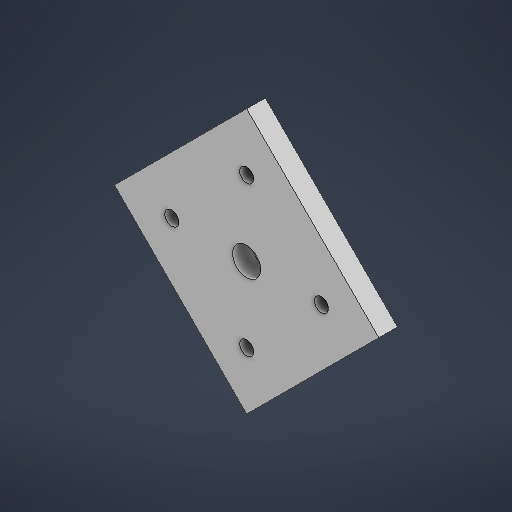
# Autodesk Inventor part: drzakmotoru_nový
Saved by Autodesk Inventor 2026 (Build 300175050, 175E)
## iProperties
Created: 2026-04-28
Part Number: drzakmotoru_nový
Material: Všeobecné
Document SubType Name: Modeling
Designer: marti
Density: 1 g/cm^3
Appearance: Výchozí
Author: marti
Autodesk Inventor part; units mm, degrees
ref_plane "YZ Plane" through (0, 0, 0) normal (1, 0, 0) x (0, 1, 0)
ref_plane "XZ Plane" through (0, 0, 0) normal (0, 1, 0) x (-1, 0, 0)
ref_plane "XY Plane" through (0, 0, 0) normal (0, 0, 1) x (1, 0, 0)
sketch "Náčrt1" plane through (0, 0, 0) normal (0, 0, 1) x (1, 0, 0)
  line L0 (-28.2843, 0) -> (0, 28.2843)
  line L1 (0, 28.2843) -> (28.2843, 0)
  line L2 (28.2843, 0) -> (0, -28.2843)
  line L3 (0, -28.2843) -> (-28.2843, 0)
  line L4 (-28.2843, 0) -> (28.2843, 0) construction
  line L5 (0, 28.2843) -> (0, -28.2843) construction
  line L6 (-28.2843, 0) -> (11.7157, 0) construction
  line L7 (0, 39.598) -> (0, -39.598) projected
  line L8 (-39.598, 0) -> (39.598, 0) projected
  point P0 (0, 0)
  point P1 (-16, 0)
  point P2 (16, 0)
  point P3 (0, 0)
  point P4 (0, 16)
  point P5 (0, -16)
  point P6 (0, 0)
  point P7 (0, 0)
  dimension "d0" = 40
  dimension "d2" = 40
  dimension "d3" = 32
  dimension "d4" = 16
  dimension "d5" = 32
  dimension "d6" = 16
  dimension "d9" = 90
  dimension "d10" = 90
  constraints: 14 end point, 4 midpoint, 4 point on line, 2 parallel, 1 coincident, 1 equal length, 1 horizontal, 1 perpendicular
  measures "d0" distance of L0.start L0.end
  measures "d2" distance of L0.end L1.end
  measures "d3" distance of point (16, 0) point (-16, 0)
  measures "d4" distance of point (16, 0) point (0, 0)
  measures "d5" distance of point (0, -16) point (0, 16)
  measures "d6" distance of point (0, 0) point (0, 16)
  measures "d9" angle of L3 L0
  measures "d10" angle of L7 L4
extrude "Vysunutí1" add sketch "Náčrt1" along normal blind 4
hole "Díra1" at (-16, 0, 0) at (16, 0, 0) at (0, 16, 0) at (0, -16, 0) direction (0, 0, 1) diameter 3 end through all
hole "Díra2" at (0, 0, 0) direction (0, 0, 1) diameter 6 end through all
equation "\"d4\" = 0.5 * d3"
equation "\"d6\" = 0.5 * d5"
